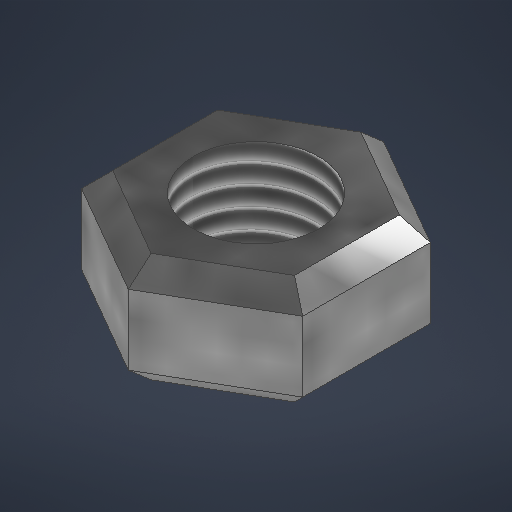
# Autodesk Inventor part: Tuerca1-4
Saved by Autodesk Inventor 2026.1 (Build 301233000, 233)
## iProperties
Created: 2026-01-17
Part Number: Tuerca1-4
Material: Genérico
Document SubType Name: Modeling
Designer: vickh
Density: 1 g/cm^3
Appearance: Acero galvanizado
Author: vickh
Autodesk Inventor part; units mm, degrees
ref_plane "YZ Plane" through (0, 0, 0) normal (1, 0, 0) x (0, 1, 0)
ref_plane "XZ Plane" through (0, 0, 0) normal (0, 1, 0) x (-1, 0, 0)
ref_plane "XY Plane" through (0, 0, 0) normal (0, 0, 1) x (1, 0, 0)
sketch "Boceto1" plane through (0, 0, 0) normal (0, 1, 0) x (-1, 0, 0)
  line L0 (0, -6.4663) -> (-5.6, -3.2332)
  line L1 (-5.6, -3.2332) -> (-5.6, 3.2332)
  line L2 (-5.6, 3.2332) -> (0, 6.4663)
  line L3 (0, 6.4663) -> (5.6, 3.2332)
  line L4 (5.6, 3.2332) -> (5.6, -3.2332)
  line L5 (5.6, -3.2332) -> (0, -6.4663)
  circle A0 centre (0, 0) radius 3.175
  line L6 (11, 0) -> (-11, 0) construction
  point P0 (2.8, -4.8497)
  point P1 (1.5875, -2.7496)
  point P2 (5.6, 0)
  dimension "d0" = 6.35
  dimension "d2" = 1.5875
  dimension "d4" = 22
  dimension "d10" = 11.2
  constraints: 14 end point, 3 coincident, 3 midpoint, 1 horizontal, 1 point on line, 16 other
  measures "d2" horizontal distance of point (0, 0) point (1.587, -2.75)
  measures "d4" distance of L6.start L6.end
  measures "d10" distance between parallel lines of L1 L4
extrude "Extrusión1" add sketch "Boceto1" along normal blind 5.55
thread "Rosca1" size "M7x1" class "6H" standard "ANSI Metric M Profile" length 60
chamfer "Chaflán1" distance 1 angle 45 12 edges at (-2.8, 5.55, 4.8497) (2.8, 5.55, 4.8497) (5.6, 5.55, 0) (2.8, 5.55, -4.8497) (-2.8, 5.55, -4.8497) (-5.6, 5.55, 0) (-5.6, 0, 0) (-2.8, 0, -4.8497) (2.8, 0, -4.8497) (5.6, 0, 0) (2.8, 0, 4.8497) (-2.8, 0, 4.8497)
